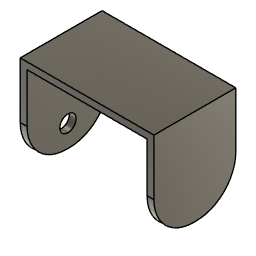
Z rotation v10 v2 (Autodesk Fusion 360 design; units mm, degrees)
Autodesk Fusion 360 part; units mm, degrees
sketch "Sketch1" plane through (0, 0, 0) normal (0, 0, 1) x (1, 0, 0)
  line L0 (-22, 15) -> (22, 15)
  line L1 (22, 15) -> (22, -15)
  line L2 (22, -15) -> (-22, -15)
  line L3 (-22, -15) -> (-22, 15)
  line L4 (-22, 15) -> (22, -15) construction
  line L5 (22, 15) -> (-22, -15) construction
  line L6 (24.5, 15) -> (22, 15)
  line L7 (22, 15) -> (22, -15)
  line L8 (22, -15) -> (24.5, -15)
  line L9 (24.5, -15) -> (24.5, 15)
  line L10 (-24.5, -15) -> (-22, -15)
  line L11 (-22, -15) -> (-22, 15)
  line L12 (-22, 15) -> (-24.5, 15)
  line L13 (-24.5, 15) -> (-24.5, -15)
  dimension "d1" = 44
  dimension "d2" = 30
  dimension "d8" = 2.5
  dimension "d9" = 2.5
  constraint horizontal L0
  constraint perpendicular L0 L1
  constraint parallel L0 L2
  constraint parallel L1 L3
  constraint coincident L4 origin
  constraint coincident L5 origin
  constraint horizontal L6
  constraint vertical L7
  constraint horizontal L8
  constraint vertical L9
  constraint coincident L0 L6.start
  constraint horizontal L10
  constraint vertical L11
  constraint horizontal L12
  constraint vertical L13
  constraint coincident L2 L10.start
  measures "d1" distance of L1.end L2.end
  measures "d2" distance of L0.end L1.end
  measures "d8" distance of L1.end L8.end
  measures "d9" distance of L10.start L2.end
extrude "Extrude1" add sketch "Sketch1" against normal blind 23 contours L3 L10 L11 L12 L13 | L1 L6 L7 L8 L9 makes body 1 at (24.5, -5, -7.6667) makes body 2 at (-22, -5, -7.6667)
extrude "Extrude2" add sketch "Sketch1" along normal blind 12 bodies 1 2
sketch "Sketch2" plane through (-24.5, 0, 0) normal (-1, 0, 0) x (0, -1, 0)
  line L0 (-15, 12) -> (-15, -23)
  line L1 (-15, -23) -> (15, -23)
  line L2 (15, -23) -> (15, 12)
  line L3 (15, 12) -> (-15, 12)
  circle A0 centre (0, -15) radius 3
  dimension "d10" = 6
  measures "d10" diameter of A0
extrude "Extrude3" cut sketch "Sketch2" against normal blind 24 contours A0 bodies 1
fillet "Fillet1" radius 14.5 4 edges at (-23.25, -15, -23) (-23.25, 15, -23) (23.25, 15, -23) (23.25, -15, -23) on bodies 1
extrude "Extrude4" cut 1 faces at (-7.3333, 5, 0) along direction (0, 0, 1) blind 9 on bodies 1 bodies 1
extrude "Extrude5" cut 1 faces at (-7.3333, 5, 9) along direction (0, 0, 1) blind 0.5 on bodies 1 bodies 1
